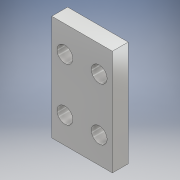
# Autodesk Inventor part: adapter_bottom
Saved by Autodesk Inventor 2018 (Build 220112000, 112)
## iProperties
Created: 2018-03-14
Part Number: adapter_bottom
Material: Générique
Document SubType Name: Modeling
Designer: Gregwar
Density: 1 g/cm^3
Appearance: Par défaut
Author: Gregwar
Autodesk Inventor part; units mm, degrees
ref_plane "YZ Plane" through (0, 0, 0) normal (1, 0, 0) x (0, 1, 0)
ref_plane "XZ Plane" through (0, 0, 0) normal (0, 1, 0) x (-1, 0, 0)
ref_plane "XY Plane" through (0, 0, 0) normal (0, 0, 1) x (1, 0, 0)
sketch "Esquisse1" plane through (0, 0, 0) normal (0, 1, 0) x (-1, 0, 0)
  line L0 (0, 0) -> (11.5, 0)
  line L1 (11.5, 0) -> (11.5, -20)
  line L2 (11.5, -20) -> (0, -20)
  line L3 (0, -20) -> (0, 0)
  line L4 (9, 0) -> (9, -20) construction
  line L5 (5.75, 0) -> (5.75, -20) construction
  line L6 (11.5, -10) -> (0, -10) construction
  circle A0 centre (9, -15) radius 1.5
  circle A1 centre (9, -5) radius 1.5
  circle A2 centre (2.5, -15) radius 1.5
  circle A3 centre (2.5, -5) radius 1.5
  dimension "d0" = 20
  dimension "d1" = 11.5
  dimension "d2" = 3
  dimension "d3" = 2.5
  dimension "d4" = 10
  constraints: 14 end point, 4 centre point, 4 midpoint, 3 point on line, 3 symmetric about line, 2 parallel, 1 horizontal, 1 perpendicular, 1 vertical, 3 other
  measures "d0" distance of L0.end L1.end
  measures "d1" distance of L0.start L0.end
  measures "d2" diameter of A0
  measures "d3" distance between parallel lines of L1 L4
  measures "d4" distance of A1.centre A0.centre
extrude "Extrusion1" add sketch "Esquisse1" along normal blind 3
sketch "Esquisse2" plane through (0, 0, 0) normal (0, -1, 0) x (1, 0, 0)
  circle A0 centre (-2.5, -5) radius 1.5 projected
  circle A1 centre (-2.5, -15) radius 1.5 projected
  circle A2 centre (-9, -5) radius 1.5 projected
  circle A3 centre (-9, -15) radius 1.5 projected
  line L0 (0, 0) -> (-11.5, 0) projected
  line L1 (-11.5, 0) -> (-11.5, -20) projected
  line L2 (-11.5, -20) -> (0, -20) projected
  line L3 (0, -20) -> (0, 0) projected
  line L4 (-11.5, 0) -> (-12, 0)
  line L5 (-12, 0) -> (-12, -20)
  line L6 (-12, -20) -> (-11.5, -20)
  line L7 (-11.5, -20) -> (-11.5, 0)
  dimension "d7" = 0.5
  constraints: 8 end point, 2 parallel, 1 horizontal, 1 perpendicular
  measures "d7" distance between parallel lines of L5 L1
extrude "Extrusion2" [suppressed]
